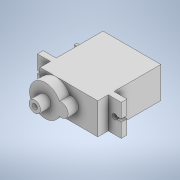
# Autodesk Inventor part: mg90s-servo
Saved by Autodesk Inventor 2021 (Build 250183000, 183)
## iProperties
Created: 2024-04-22
Part Number: mg90s-servo
Material: Generic
Document SubType Name: Modeling
Designer: Toby
Density: 1 g/cm^3
Appearance: Default
Author: Toby
Autodesk Inventor part; units mm, degrees
ref_plane "YZ Plane" through (0, 0, 0) normal (1, 0, 0) x (0, 1, 0)
ref_plane "XZ Plane" through (0, 0, 0) normal (0, 1, 0) x (-1, 0, 0)
ref_plane "XY Plane" through (0, 0, 0) normal (0, 0, 1) x (1, 0, 0)
sketch "Sketch1" plane through (0, 0, 0) normal (0, 0, 1) x (1, 0, 0)
  line L0 (-11.1, 6) -> (11.1, 6)
  line L1 (11.1, 6) -> (11.1, -6)
  line L2 (11.1, -6) -> (-11.1, -6)
  line L3 (-11.1, -6) -> (-11.1, 6)
  point P0 (0, 0)
  dimension "d0" = 22.2
  dimension "d1" = 12
  dimension "d2" = 6
  dimension "d3" = 11.1
  constraints: 8 end point, 2 parallel, 1 horizontal, 1 perpendicular
  measures "d0" distance of L0.start L0.end
  measures "d1" distance of L2.end L0.start
  measures "d2" distance from line of point (0, 0) L0
  measures "d3" distance from line of point (0, 0) L3
extrude "Extrusion1" add sketch "Sketch1" along normal blind 18
sketch "Sketch2" plane through (0, 0, 18) normal (0, 0, 1) x (1, 0, 0)
  line L0 (-16.1, 6) -> (16.1, 6)
  line L1 (16.1, 6) -> (16.1, -6)
  line L2 (16.1, -6) -> (-16.1, -6)
  line L3 (-16.1, -6) -> (-16.1, 6)
  line L4 (11.1, 6) -> (-11.1, 6) projected
  line L5 (-11.1, -6) -> (11.1, -6) projected
  line L6 (-11.1, 6) -> (-11.1, -6) projected
  line L7 (11.1, -6) -> (11.1, 6) projected
  point P0 (0, 0)
  dimension "d6" = 5
  dimension "d7" = 5
  constraints: 8 end point, 2 collinear, 2 parallel, 1 horizontal, 1 perpendicular
  measures "d6" distance between parallel lines of L6 L3
  measures "d7" distance between parallel lines of L7 L1
extrude "Extrusion2" add sketch "Sketch2" along normal blind 2.2
sketch "Sketch3" plane through (0, 0, 20.2) normal (0, 0, 1) x (1, 0, 0)
  line L0 (16.1, 6) -> (-16.1, 6) projected
  line L1 (-16.1, -6) -> (16.1, -6) projected
  line L2 (-11.1, 6) -> (11.1, 6)
  line L3 (11.1, 6) -> (11.1, -6)
  line L4 (11.1, -6) -> (-11.1, -6)
  line L5 (-11.1, -6) -> (-11.1, 6)
  line L6 (-16.1, 6) -> (-16.1, -6) projected
  line L7 (16.1, -6) -> (16.1, 6) projected
  point P0 (0, 0)
  point P1 (-11.1, -6)
  dimension "d10" = 5
  dimension "d11" = 5
  constraints: 8 end point, 2 parallel, 2 point on line, 1 horizontal, 1 perpendicular
  measures "d10" distance between parallel lines of L6 L5
  measures "d11" distance between parallel lines of L7 L3
extrude "Extrusion3" add sketch "Sketch3" along normal blind 4 contours L3 L1 L5 L0
sketch "Sketch4" plane through (0, 0, 24.2) normal (0, 0, 1) x (1, 0, 0)
  circle A0 centre (-5.1, 0) radius 6
  line L0 (11.1, 6) -> (-11.1, 6) projected
  line L1 (-11.1, 6) -> (-11.1, -6) projected
  point P0 (0, 0)
  dimension "d14" = 6
  constraints: 1 centre point, 1 tangent
  measures "d14" distance from line of L1 A0.centre
extrude "Extrusion4" add sketch "Sketch4" along normal blind 4 contours A0
sketch "Sketch5" plane through (0, 0, 24.2) normal (0, 0, 1) x (1, 0, 0)
  circle A0 centre (1.1, 0) radius 2.6
  line L0 (11.1, -6) -> (11.1, 6) projected
  point P0 (0, 0)
  dimension "d17" = 5.2
  dimension "d18" = 10
  constraints: 1 centre point
  measures "d17" diameter of A0
  measures "d18" distance from line of A0.centre L0
extrude "Extrusion5" add sketch "Sketch5" along normal blind 4
sketch "Sketch6" plane through (0, 0, 28.2) normal (0, 0, 1) x (1, 0, 0)
  arc A0 (0.3581, 2.4919) -> (0.3581, -2.4919) centre (-5.1, 0) ccw projected
  circle A1 centre (-5.1, 0) radius 2.2
  point P0 (0, 0)
  dimension "d21" = 4.4
  constraints: 1 centre point, 1 coincident
  measures "d21" diameter of A1
extrude "Extrusion6" add sketch "Sketch6" along normal blind 4
sketch "Sketch7" plane through (-5.1, 0, 32.2) normal (0, 0, 1) x (1, 0, 0)
  point P0 (5.1, 0)
  point P1 (0, 0)
hole "Hole1" at (-5.1, 0, 32.2) direction (0, 0, -1) diameter 2 depth 4 tip angle 118
sketch "Sketch8" plane through (0, 0, 20.2) normal (0, 0, 1) x (1, 0, 0)
  line L0 (-16.1, 6) -> (-16.1, -6) projected
  line L1 (16.1, -6) -> (16.1, 6) projected
  point P0 (0, 0)
  point P1 (-13.6, 0)
  point P2 (13.6, 0)
  dimension "d31" = 2.5
  dimension "d32" = 2.5
  measures "d31" distance from line of L0 point (-13.6, 0)
  measures "d32" distance from line of L1 point (13.6, 0)
hole "Hole2" at (-13.6, 0, 20.2) at (13.6, 0, 20.2) direction (0, 0, -1) diameter 2 depth 4 tip angle 118
sketch "Sketch9" plane through (0, 0, 20.2) normal (0, 0, 1) x (1, 0, 0)
  line L0 (-16.1, 6) -> (-16.1, -6) projected
  line L1 (-16.1, 0.5) -> (-14.0089, 0.5)
  line L2 (-14.0089, 0.5) -> (-14.0089, -0.5)
  line L3 (-14.0089, -0.5) -> (-16.1, -0.5)
  line L4 (-16.1, -0.5) -> (-16.1, 0.5)
  circle A0 centre (-13.6, 0) radius 1 projected
  line L5 (16.1, -6) -> (16.1, 6) projected
  line L6 (13.947, 0.5) -> (16.1, 0.5)
  line L7 (16.1, 0.5) -> (16.1, -0.5)
  line L8 (16.1, -0.5) -> (13.947, -0.5)
  line L9 (13.947, -0.5) -> (13.947, 0.5)
  circle A1 centre (13.6, 0) radius 1 projected
  point P0 (0, 0)
  point P1 (-14.466, -0.5)
  point P2 (-14.466, 0.5)
  dimension "d40" = 1
  dimension "d41" = 0.5
  dimension "d42" = 1
  dimension "d43" = 0.5
  constraints: 16 end point, 4 parallel, 2 horizontal, 2 perpendicular, 2 point on line
  measures "d40" distance between parallel lines of L3 L1
  measures "d41" distance from line of A0.centre L1
  measures "d42" distance between parallel lines of L8 L6
  measures "d43" distance centre to line of A1 L6
extrude "Extrusion7" cut sketch "Sketch9" against normal blind 4 contours L1 A0 L3 L0 | L8 A1 L6 L5 | L8 L9 L6 A1 picked at (14.1647, 0)
sketch "Sketch10" plane through (-11.1, -6, 0) normal (-1, 0, 0) x (0, 0, 1)
  line L0 (6, 8) -> (5, 8)
  line L1 (5, 8) -> (5, 4)
  line L2 (5, 4) -> (6, 4)
  line L3 (6, 4) -> (6, 8)
  line L4 (0, 12) -> (0, 0) projected
  line L5 (0, 0) -> (18, 0) projected
  line L6 (0, 12) -> (18, 12) projected
  point P0 (0, 6)
  dimension "d46" = 1
  dimension "d47" = 5
  dimension "d48" = 4
  dimension "d49" = 4
  constraints: 8 end point, 2 parallel, 1 horizontal, 1 perpendicular
  measures "d46" distance between parallel lines of L1 L3
  measures "d47" distance between parallel lines of L4 L1
  measures "d48" distance between parallel lines of L5 L2
  measures "d49" distance between parallel lines of L6 L0
extrude "Extrusion8" add sketch "Sketch10" along normal blind 5
body "Solid1"
